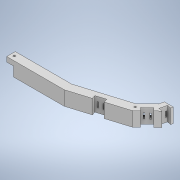
# Autodesk Inventor part: bumper_base_final _원본수정
Saved by Autodesk Inventor 2020 (Build 240168000, 168)
## iProperties
Created: 2022-06-30
Part Number: bumper_base_final _원본수정
Material: 일반
Document SubType Name: Modeling
Designer: samsung
Density: 1 g/cm^3
Appearance: 기본값
Author: samsung
Autodesk Inventor part; units mm, degrees
ref_plane "YZ Plane" through (0, 0, 0) normal (1, 0, 0) x (0, 1, 0)
ref_plane "XZ Plane" through (0, 0, 0) normal (0, 1, 0) x (-1, 0, 0)
ref_plane "XY Plane" through (0, 0, 0) normal (0, 0, 1) x (1, 0, 0)
sketch "스케치1" plane through (0, 0, 0) normal (0, 1, 0) x (-1, 0, 0)
  line L0 (-417.5, 136.0278) -> (167.5, 136.0278)
  arc A0 (156.6099, 73.7155) -> (-406.6899, 73.6783) centre (-125, -531.4722) ccw
  arc A1 (148.4052, 66.4876) -> (-398.3844, 66.4971) centre (-125, -531.4722) ccw
  line L1 (143.8982, 68.5278) -> (-85, 68.5278)
  line L2 (-165, 68.5278) -> (-393.8982, 68.5278)
  line L3 (-125, -531.4722) -> (-125, 1435.9267)
  circle A2 centre (-125, -531.4722) radius 1967.3989
  line L4 (-125, 111.6599) -> (-436.953, 1411.0375)
  line L5 (-125, 111.6599) -> (186.953, 1411.0375)
  line L6 (-417.5444, 28.5399) -> (-406.6899, 73.6783)
  line L7 (-407.5098, 28.5399) -> (-398.3801, 66.5058)
  arc A3 (1441.9544, 38.2515) -> (-1691.7763, 38.7413) centre (-125, -531.4722) ccw
  line L8 (-371.3038, 78.1512) -> (-261.7019, 111.6599)
  line L9 (-261.7019, 111.6599) -> (11.7019, 111.6599)
  line L10 (-316.5029, 94.9056) -> (-320.1581, 106.8613)
  line L11 (-316.5029, 94.9056) -> (-397.3646, 1416.9826)
  line L12 (-316.5029, 94.9056) -> (-988.7616, 1236.1743)
  line L13 (-398.3844, 66.4971) -> (-125, -531.4722)
  line L14 (-407.5098, 28.5399) -> (-405.1717, 38.2627)
  line L15 (-405.1717, 38.2627) -> (-414.6578, 40.5439)
  line L16 (-405.1717, 38.2627) -> (-1671.8283, 684.2501)
  line L17 (-405.1717, 38.2627) -> (-2007.9181, 38.8589)
  line L18 (-405.1717, 38.2627) -> (-402.8337, 47.9856)
  line L19 (-402.8337, 47.9856) -> (-371.3038, 78.1512)
  line L20 (-387.0687, 63.0684) -> (-400.1089, 76.6983)
  line L21 (-387.0687, 63.0684) -> (-1557.9022, 816.656)
  line L22 (-387.0687, 63.0684) -> (-1051.9279, 1203.8846)
  line L23 (-125, -531.4722) -> (-261.7019, 111.6599)
  line L24 (-125, -531.4722) -> (11.7019, 111.6599)
  line L25 (-417.5444, 28.5399) -> (-407.5098, 28.5399)
  line L26 (-125, -531.4722) -> (-371.3038, 78.1512)
  line L27 (-125, -531.4722) -> (121.3038, 78.1512)
  line L28 (11.7019, 111.6599) -> (121.3038, 78.1512)
  line L29 (167.4556, 28.5399) -> (156.6099, 73.7155)
  line L30 (157.5156, 28.5399) -> (148.4052, 66.4876)
  line L31 (121.3038, 78.1512) -> (152.8486, 47.9794)
  line L32 (155.1841, 38.2515) -> (1758.102, 38.2515)
  line L33 (155.1841, 38.2515) -> (164.5823, 40.5079)
  line L34 (157.5156, 28.5399) -> (167.4556, 28.5399)
  line L35 (155.1841, 38.2515) -> (1422.1711, 683.8137)
  line L36 (66.5029, 94.9056) -> (70.1581, 106.8613)
  line L37 (66.5029, 94.9056) -> (738.7616, 1236.1743)
  line L38 (66.5029, 94.9056) -> (147.3646, 1416.9826)
  line L39 (137.0762, 63.0653) -> (150.1137, 76.6961)
  line L40 (137.0762, 63.0653) -> (801.7772, 1203.965)
  line L41 (137.0762, 63.0653) -> (1307.7755, 816.7906)
  line L42 (-125, -531.4722) -> (148.4052, 66.4876)
  line L43 (-259.0118, 93.6599) -> (9.0118, 93.6599)
  line L44 (111.9521, 62.1879) -> (136.5817, 38.6304)
  line L45 (9.0118, 93.6599) -> (111.9521, 62.1879)
  line L46 (-361.9509, 62.1883) -> (-386.641, 38.5664)
  line L47 (-387.0049, 38.256) -> (-387.0101, 38.2515)
  line L48 (-388.9967, 28.5399) -> (-386.569, 38.6353)
  line L49 (-361.9509, 62.1883) -> (-259.0118, 93.6599)
  line L50 (-407.5098, 28.5399) -> (-388.9967, 28.5399)
  line L51 (136.5817, 38.6304) -> (139.0042, 28.5399)
  line L52 (157.5156, 28.5399) -> (139.0042, 28.5399)
  line L53 (-125, 111.6599) -> (-155, 111.6599)
  line L54 (-155, 93.6599) -> (-125, 93.6599)
  line L55 (-125, 93.6599) -> (-125, 111.6599)
  line L56 (-155, 93.6599) -> (-155, 111.6599)
  line L57 (-135, 111.6599) -> (-135, 93.6599)
  line L58 (-141, 111.6599) -> (-141, 93.6599)
  point P0 (0, 0)
  point P1 (0, 0)
  point P2 (143.8982, 61.5)
  point P3 (-393.8982, 61.5)
  point P4 (-417.5, 21.5)
  point P5 (-165, 0)
  point P6 (-85, 0)
  point P7 (-85, 12.4229)
  point P8 (167.5, 12.4229)
  point P9 (-393.8982, -388.5)
  point P10 (-165, -388.5)
  point P11 (167.5, -327)
  point P12 (-417.5, -327)
  point P13 (-85, -388.5)
  point P14 (143.8982, -388.5)
  point P15 (162, 21.5)
  point P16 (162, 12.4229)
  point P17 (167.5, 21.5)
  point P18 (-125, 0)
  point P19 (-125, 136.0278)
  point P20 (-125, 136.0278)
  point P21 (-125, 93.6599)
  point P22 (-148, 102.6599)
  dimension "d12" = 657.5
  dimension "d13" = 667.5
  dimension "d15" = 585
  dimension "d25" = 1299.8989
  dimension "d30" = 13.5
  dimension "d31" = 13.5
  dimension "d39" = 999.8126
  dimension "d45" = 13.5
  dimension "d46" = 13.5
  dimension "d50" = 10
  dimension "d51" = 13.5
  dimension "d52" = 13.5
  dimension "d53" = 10
  dimension "d54" = 13.5
  dimension "d55" = 13.5
  dimension "d56" = 12
  dimension "d57" = 12
  dimension "d60" = 10
  dimension "d65" = 13.5
  dimension "d66" = 13.5
  dimension "d68" = 13.5
  dimension "d69" = 13.5
  dimension "d70" = 13.5
  dimension "d71" = 13.5
  dimension "d72" = 10
  dimension "d83" = 18
  dimension "d84" = 18
  dimension "d85" = 18
  dimension "d86" = 18
  dimension "d212" = 18
  dimension "d213" = 30
  dimension "d214" = 7
  dimension "d215" = 10
  dimension "d216" = 14
  dimension "d218" = 9
  constraints: 118 end point, 18 point on line, 17 point on circle, 8 horizontal, 8 parallel, 7 perpendicular, 6 midpoint, 3 centre point, 2 vertical, 1 coincident, 1 tangent, 18 other
  measures "d12" radius of A1
  measures "d13" radius of A0
  measures "d15" distance of L29.start L6.start
  measures "d30" angle of L4 L3
  measures "d31" angle of L5 L3
  measures "d39" radial gap between concentric circles of A0 A3
  measures "d45" angle of L10 L11
  measures "d46" angle of L12 L10
  measures "d50" distance of L7.start L14.end
  measures "d51" angle of L16 L15
  measures "d52" angle of L17 L15
  measures "d53" distance of L14.end L18.end
  measures "d54" angle of L20 L22
  measures "d55" angle of L20 L21
  measures "d56" angle of L3 L23
  measures "d57" angle of L24 L3
  measures "d60" angle of L26 L23
  measures "d65" angle of L33 L32
  measures "d66" angle of L35 L33
  measures "d68" angle of L37 L36
  measures "d69" angle of L36 L38
  measures "d70" angle of L40 L39
  measures "d71" angle of L41 L39
  measures "d72" angle of L27 L24
  measures "d83" distance between parallel lines of L31 L44
  measures "d84" distance between parallel lines of L19 L46
  measures "d85" distance between parallel lines of L14 L48
  measures "d86" distance between parallel lines of L30 L51
  measures "d212" distance of L54.end L4.start
  measures "d213" distance of L54.start L54.end
  measures "d214" distance from line of L56 point (-148, 102.66)
  measures "d215" distance between parallel lines of L57 L55
  measures "d216" distance between parallel lines of L56 L58
  measures "d218" distance from line of L54 point (-148, 102.66)
extrude "돌출11" add sketch "스케치1" against normal blind 30 contours L26 L2 L19 | L8 L23 L43 L49 L2 L26 | L9 L56 L43 L23 | L2 L26 L46 L13 L19 | L2 L49 L46 L26 | L9 L58 L43 L56 | L13 L46 L48 L50 L7 L19
sketch "스케치14" plane through (141, 0, 93.6599) normal (-1, 0, 0) x (0, 0, 1)
  line L0 (0, 0) -> (18, 0) projected
  line L1 (0, 0) -> (0, -30) projected
  line L2 (18, -30) -> (0, -30) projected
  line L3 (18, 0) -> (18, -30) projected
  line L4 (0, -10) -> (18, -10)
  point P0 (-93.6599, 0)
  dimension "d161" = 20
  constraints: 2 end point, 2 point on line, 1 perpendicular
  measures "d161" distance between parallel lines of L2 L4
extrude "돌출12" cut sketch "스케치14" against normal blind 14 contours L4 L3 L2 L1
sketch "스케치15" plane through (261.7019, -30, 111.6599) normal (0.2923717, 0, 0.9563048) x (0.9563048, 0, -0.2923717)
  line L0 (0, 30) -> (114.6098, 30) projected
  line L1 (0, 30) -> (0, 0) projected
  line L2 (114.6098, 0) -> (0, 0) projected
  line L3 (114.6098, 30) -> (114.6098, 0) projected
  line L4 (114.6098, 0) -> (0, 0) projected
  line L5 (47.3049, 30) -> (67.3049, 30)
  line L6 (67.3049, 30) -> (67.3049, 0)
  line L7 (67.3049, 0) -> (47.3049, 0)
  line L8 (47.3049, 0) -> (47.3049, 30)
  line L9 (47.3049, 30) -> (67.3049, 0) construction
  line L10 (67.3049, 30) -> (47.3049, 0) construction
  point P0 (-217.6206, 30)
  point P1 (57.3049, 15)
  dimension "d164" = 20
  constraints: 12 end point, 2 midpoint, 2 parallel, 1 horizontal, 1 perpendicular, 1 point on line
  measures "d164" distance of L6.end L7.end
extrude "돌출13" cut sketch "스케치15" against normal blind 8 contours L0 L6 L2 L8
sketch "스케치16" plane through (259.363, -30, 104.0094) normal (0.2923717, 0, 0.9563048) x (0.9563048, 0, -0.2923717)
  line L0 (67.3049, 0) -> (47.3049, 0) projected
  line L1 (67.3049, 30) -> (67.3049, 0) projected
  line L2 (47.3049, 30) -> (67.3049, 30) projected
  line L3 (47.3049, 0) -> (47.3049, 30) projected
  line L4 (52.3049, 20.5) -> (62.3049, 20.5)
  line L5 (62.3049, 20.5) -> (62.3049, 9.5)
  line L6 (62.3049, 9.5) -> (52.3049, 9.5)
  line L7 (52.3049, 9.5) -> (52.3049, 20.5)
  line L8 (52.3049, 20.5) -> (62.3049, 9.5) construction
  line L9 (62.3049, 20.5) -> (52.3049, 9.5) construction
  line L10 (61.0549, 20.5) -> (63.5549, 20.5)
  line L11 (63.5549, 20.5) -> (63.5549, 9.5)
  line L12 (63.5549, 9.5) -> (61.0549, 9.5)
  line L13 (61.0549, 9.5) -> (61.0549, 20.5)
  line L14 (61.0549, 20.5) -> (63.5549, 9.5) construction
  line L15 (63.5549, 20.5) -> (61.0549, 9.5) construction
  line L16 (51.0549, 20.5) -> (53.5549, 20.5)
  line L17 (53.5549, 20.5) -> (53.5549, 9.5)
  line L18 (53.5549, 9.5) -> (51.0549, 9.5)
  line L19 (51.0549, 9.5) -> (51.0549, 20.5)
  line L20 (51.0549, 20.5) -> (53.5549, 9.5) construction
  line L21 (53.5549, 20.5) -> (51.0549, 9.5) construction
  point P0 (-217.6206, 30)
  point P1 (57.3049, 15)
  point P2 (62.3049, 15)
  point P3 (52.3049, 15)
  point P4 (57.3049, 15)
  point P5 (57.3049, 30)
  point P6 (57.3049, 15)
  point P7 (47.3049, 15)
  point P8 (61.0549, 20.5)
  point P9 (61.0549, 9.5)
  point P10 (62.3049, 9.5)
  point P11 (52.3049, 9.5)
  point P12 (53.5549, 20.5)
  point P13 (52.3049, 20.5)
  dimension "d167" = 10
  dimension "d168" = 11
  dimension "d169" = 2.5
  dimension "d170" = 2.5
  constraints: 36 end point, 13 midpoint, 6 parallel, 3 horizontal, 3 perpendicular, 1 horizontal alignment, 1 point on line, 1 vertical alignment
  measures "d167" distance of L5.end L6.end
  measures "d168" distance of L4.end L5.end
  measures "d169" distance of L11.end L12.end
  measures "d170" distance of L17.end L18.end
extrude "돌출14" cut sketch "스케치16" against normal blind 10 contours L4 L17 L6 L7 | L7 L18 L19 L16 | L4 L5 L6 L13 | L10 L11 L12 L5
sketch "스케치17" plane through (371.3038, -30, 78.1512) normal (0.6913026, 0, 0.7225653) x (0.7225653, 0, -0.6913026)
  line L0 (0, 30) -> (43.636, 30) projected
  line L1 (0, 30) -> (0, 0) projected
  line L2 (43.636, 0) -> (0, 0) projected
  line L3 (43.636, 30) -> (43.636, 0) projected
  line L4 (11.818, 30) -> (31.818, 30)
  line L5 (31.818, 30) -> (31.818, 0)
  line L6 (31.818, 0) -> (11.818, 0)
  line L7 (11.818, 0) -> (11.818, 30)
  line L8 (11.818, 30) -> (31.818, 0) construction
  line L9 (31.818, 30) -> (11.818, 0) construction
  point P0 (-214.2651, 30)
  point P1 (21.818, 15)
  point P2 (11.818, 30)
  point P3 (11.818, 0)
  point P4 (31.818, 0)
  point P5 (31.818, 30)
  dimension "d173" = 20
  dimension "d174" = 30
  constraints: 12 end point, 2 midpoint, 2 parallel, 1 horizontal, 1 perpendicular
  measures "d173" distance of L5.end L6.end
  measures "d174" distance of L4.end L5.end
extrude "돌출15" cut sketch "스케치17" against normal blind 8 contours L0 L5 L2 L7
sketch "스케치18" plane through (365.7734, -30, 72.3707) normal (0.6913026, 0, 0.7225653) x (0.7225653, 0, -0.6913026)
  line L0 (11.818, 0) -> (11.818, 30) projected
  line L1 (31.818, 0) -> (11.818, 0) projected
  line L2 (31.818, 30) -> (31.818, 0) projected
  line L3 (11.818, 30) -> (31.818, 30) projected
  line L4 (16.818, 20.5) -> (26.818, 20.5)
  line L5 (26.818, 20.5) -> (26.818, 9.5)
  line L6 (26.818, 9.5) -> (16.818, 9.5)
  line L7 (16.818, 9.5) -> (16.818, 20.5)
  line L8 (16.818, 20.5) -> (26.818, 9.5) construction
  line L9 (26.818, 20.5) -> (16.818, 9.5) construction
  line L10 (25.568, 20.5) -> (28.068, 20.5)
  line L11 (28.068, 20.5) -> (28.068, 9.5)
  line L12 (28.068, 9.5) -> (25.568, 9.5)
  line L13 (25.568, 9.5) -> (25.568, 20.5)
  line L14 (25.568, 20.5) -> (28.068, 9.5) construction
  line L15 (28.068, 20.5) -> (25.568, 9.5) construction
  line L16 (15.568, 20.5) -> (18.068, 20.5)
  line L17 (18.068, 20.5) -> (18.068, 9.5)
  line L18 (18.068, 9.5) -> (15.568, 9.5)
  line L19 (15.568, 9.5) -> (15.568, 20.5)
  line L20 (15.568, 20.5) -> (18.068, 9.5) construction
  line L21 (18.068, 20.5) -> (15.568, 9.5) construction
  point P0 (-214.2651, 30)
  point P1 (21.818, 15)
  point P2 (26.818, 15)
  point P3 (16.818, 15)
  point P4 (21.818, 15)
  point P5 (21.818, 30)
  point P6 (21.818, 15)
  point P7 (11.818, 15)
  point P8 (25.568, 20.5)
  point P9 (25.568, 9.5)
  point P10 (26.818, 9.5)
  point P11 (18.068, 20.5)
  point P12 (16.818, 20.5)
  point P13 (16.818, 9.5)
  dimension "d177" = 10
  dimension "d178" = 11
  dimension "d179" = 2.5
  dimension "d180" = 2.5
  constraints: 36 end point, 13 midpoint, 6 parallel, 3 horizontal, 3 perpendicular, 1 horizontal alignment, 1 point on line, 1 vertical alignment
  measures "d177" distance of L5.end L6.end
  measures "d178" distance of L4.end L5.end
  measures "d179" distance of L11.end L12.end
  measures "d180" distance of L17.end L18.end
extrude "돌출16" cut sketch "스케치18" against normal blind 10 contours L4 L17 L6 L7 | L7 L18 L19 L16 | L4 L5 L6 L13 | L10 L11 L12 L5
sketch "스케치19" plane through (402.8337, -30, 47.9856) normal (0.972283, 0, 0.233807) x (0.233807, 0, -0.972283)
  line L0 (15.6715, 30) -> (15.6715, 0) projected
  line L1 (0, 30) -> (20, 30) projected
  line L2 (0, 30) -> (0, 0) projected
  line L3 (20, 0) -> (0, 0) projected
  line L4 (20, 30) -> (20, 0) projected
  line L5 (5.2884, 0) -> (15.6715, 0) projected
  line L6 (0, 30) -> (15, 30)
  line L7 (15, 30) -> (15, 0)
  line L8 (15, 0) -> (0, 0)
  line L9 (0, 0) -> (0, 30)
  point P0 (-47.5298, 30)
  point P1 (15, 0)
  point P2 (15, 30)
  dimension "d183" = 15
  constraints: 8 end point, 2 parallel, 1 horizontal, 1 perpendicular, 1 point on line
  measures "d183" distance of L7.end L8.end
extrude "돌출17" cut sketch "스케치19" against normal blind 8 contours L7 L3 L2 L1
sketch "스케치20" plane through (395.0554, -30, 46.1151) normal (0.972283, 0, 0.233807) x (0.233807, 0, -0.972283)
  line L0 (15, 0) -> (0, 0) projected
  line L1 (15, 30) -> (15, 0) projected
  line L2 (0, 30) -> (15, 30) projected
  line L3 (0, 0) -> (0, 30) projected
  line L4 (2.5, 20.5) -> (12.5, 20.5)
  line L5 (12.5, 20.5) -> (12.5, 9.5)
  line L6 (12.5, 9.5) -> (2.5, 9.5)
  line L7 (2.5, 9.5) -> (2.5, 20.5)
  line L8 (2.5, 20.5) -> (12.5, 9.5) construction
  line L9 (12.5, 20.5) -> (2.5, 9.5) construction
  line L10 (11.25, 20.5) -> (13.75, 20.5)
  line L11 (13.75, 20.5) -> (13.75, 9.5)
  line L12 (13.75, 9.5) -> (11.25, 9.5)
  line L13 (11.25, 9.5) -> (11.25, 20.5)
  line L14 (11.25, 20.5) -> (13.75, 9.5) construction
  line L15 (13.75, 20.5) -> (11.25, 9.5) construction
  line L16 (1.25, 20.5) -> (3.75, 20.5)
  line L17 (3.75, 20.5) -> (3.75, 9.5)
  line L18 (3.75, 9.5) -> (1.25, 9.5)
  line L19 (1.25, 9.5) -> (1.25, 20.5)
  line L20 (1.25, 20.5) -> (3.75, 9.5) construction
  line L21 (3.75, 20.5) -> (1.25, 9.5) construction
  point P0 (-47.5298, 30)
  point P1 (7.5, 15)
  point P2 (12.5, 15)
  point P3 (2.5, 15)
  point P4 (2.5, 9.5)
  point P5 (11.25, 20.5)
  point P6 (11.25, 9.5)
  point P7 (12.5, 9.5)
  dimension "d186" = 10
  dimension "d187" = 11
  dimension "d188" = 2.5
  dimension "d189" = 2.5
  constraints: 36 end point, 8 midpoint, 6 parallel, 3 horizontal, 3 perpendicular, 2 point on line
  measures "d186" distance of L5.end L6.end
  measures "d187" distance of L4.end L5.end
  measures "d188" distance of L11.end L12.end
  measures "d189" distance of L17.end L18.end
extrude "돌출18" cut sketch "스케치20" against normal through all contours L4 L17 L6 L7 | L7 L18 L19 L16 | L4 L5 L6 L13 | L10 L11 L12 L5
sketch "스케치21" plane through (0, -30, 0) normal (0, -1, 0) x (1, 0, 0)
  line L0 (388.9967, 28.5399) -> (407.5098, 28.5399) projected
  point P0 (0, 0)
  point P1 (367.5098, 68.5399)
  dimension "d192" = 40
  dimension "d193" = 40
  measures "d192" distance from line of L0 point (367.51, 68.54)
  measures "d193" horizontal distance of point (367.51, 68.54) L0.end
hole "구멍3" at (367.5098, -30, 68.5399) direction (0, 1, 0) diameter 4.2 end through all counterbore diameter 8 counterbore depth 15
sketch "스케치22" plane through (0, 0, 0) normal (0, 1, 0) x (1, 0, 0)
  circle A0 centre (367.5098, -68.5399) radius 2.1 projected
  line L0 (402.8337, -47.9856) -> (395.0554, -46.1151) projected
  line L1 (395.0554, -46.1151) -> (398.5625, -31.5309) projected
  line L2 (398.5625, -31.5309) -> (406.3408, -33.4013) projected
  line L3 (406.3408, -33.4013) -> (407.5098, -28.5399) projected
  line L4 (407.5098, -28.5399) -> (388.9967, -28.5399) projected
  line L5 (388.9967, -28.5399) -> (386.569, -38.6353) projected
  line L6 (386.569, -38.6353) -> (361.9509, -62.1883) projected
  line L7 (361.9509, -62.1883) -> (259.0118, -93.6599) projected
  line L8 (259.0118, -93.6599) -> (141, -93.6599) projected
  line L9 (141, -111.6599) -> (261.7019, -111.6599) projected
  line L10 (261.7019, -111.6599) -> (306.9398, -97.8293) projected
  line L11 (306.9398, -97.8293) -> (304.6009, -90.1788) projected
  line L12 (304.6009, -90.1788) -> (323.727, -84.3314) projected
  line L13 (323.727, -84.3314) -> (326.0659, -91.9818) projected
  line L14 (326.0659, -91.9818) -> (371.3038, -78.1512) projected
  line L15 (371.3038, -78.1512) -> (379.8431, -69.9814) projected
  line L16 (379.8431, -69.9814) -> (374.3127, -64.2009) projected
  line L17 (374.3127, -64.2009) -> (388.764, -50.3749) projected
  line L18 (388.764, -50.3749) -> (394.2944, -56.1554) projected
  line L19 (394.2944, -56.1554) -> (402.8337, -47.9856) projected
  line L20 (141, -93.6599) -> (141, -111.6599) projected
  point P0 (0, 0)
  point P1 (148, -102.6599)
  dimension "d202" = 9
  dimension "d217" = 7
  measures "d202" distance from line of point (148, -102.66) L9
  measures "d217" distance from line of L20 point (148, -102.66)
hole "구멍4" at (148, 0, 102.6599) direction (0, -1, 0) diameter 4.2 end through all
equation "\"d46\" = d45"
equation "\"d57\" = d56"
equation "\"d72\" = d60"
equation "\"d61\" = d60"
